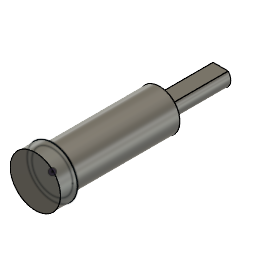
Rear axcel (Autodesk Fusion 360 design; units mm, degrees)
Autodesk Fusion 360 part; units mm, degrees
sketch "Sketch1" plane through (0, 0, 0) normal (0, 0, 1) x (1, 0, 0)
  circle A0 centre (0, 0) radius 3
  circle A1 centre (0, 0) radius 3.7
  dimension "d1" = 6
  dimension "d2" = 7.4
  constraint coincident A0.centre A1.centre
  constraint concentric A0 A1
  measures "d1" diameter of A0
  measures "d2" diameter of A1
extrude "Extrude1" add sketch "Sketch1" along normal blind 2.5 contours A0 | A1
extrude "Extrude2" add sketch "Sketch1" against normal blind 15.8 contours A0
sketch "Sketch2" plane through (0, 0, -15.8) normal (0, 0, -1) x (-1, 0, 0)
  circle A0 centre (0, 0) radius 3
  circle A1 centre (0, 0) radius 1.5
  line L0 (-2.2147, 1) -> (2, 1)
  dimension "d7" = 3
  dimension "d8" = 1
  constraint coincident A0.centre A1.centre
  constraint horizontal L0
  measures "d7" diameter of A1
  measures "d8" distance of A0.centre L0
extrude "Extrude3" add sketch "Sketch2" along normal blind 9 contours A1 L0 picked at (0.3583, 0.0454)
